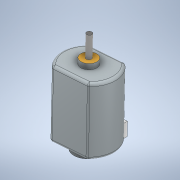
# Autodesk Inventor part: motor
Saved by Autodesk Inventor 2022 (Build 260153000, 153)
## iProperties
Created: 2022-06-21
Part Number: motor
Material: Generisch
Document SubType Name: Modeling
Designer: Friedrich Walmrath
Density: 1 g/cm^3
Appearance: Zink
Author: Friedrich Walmrath
Autodesk Inventor part; units mm, degrees
ref_plane "YZ Plane" through (0, 0, 0) normal (1, 0, 0) x (0, 1, 0)
ref_plane "XZ Plane" through (0, 0, 0) normal (0, 1, 0) x (-1, 0, 0)
ref_plane "XY Plane" through (0, 0, 0) normal (0, 0, 1) x (1, 0, 0)
sketch "Skizze1" plane through (0, 0, 0) normal (0, 0, 1) x (1, 0, 0)
  circle A0 centre (0, 0) radius 10
  line L0 (-6.6144, 7.5) -> (6.6144, 7.5)
  line L1 (-6.6144, -7.5) -> (6.6144, -7.5)
  dimension "d0" = 20
  dimension "d1" = 15
  constraints: 4 end point, 4 point on circle, 2 vertical alignment, 1 centre point, 1 coincident, 1 horizontal, 1 parallel
  measures "d0" diameter of A0
  measures "d1" distance between parallel lines of L1 L0
extrude "Extrusion1" add sketch "Skizze1" along normal blind 25 contours A0 L1 L0
sketch "Skizze2" plane through (0, 0, 25) normal (0, 0, 1) x (1, 0, 0)
  circle A0 centre (0, 0) radius 3
  dimension "d5" = 6
  constraints: 1 centre point, 1 coincident
  measures "d5" diameter of A0
extrude "Extrusion2" add sketch "Skizze2" along normal blind 2
sketch "Skizze3" plane through (0, 0, 27) normal (0, 0, 1) x (1, 0, 0)
  circle A0 centre (0, 0) radius 1
  dimension "d8" = 2
  constraints: 1 centre point, 1 coincident
  measures "d8" diameter of A0
extrude "Extrusion3" add sketch "Skizze3" along normal blind 8
sketch "Skizze5" plane through (-6.6144, 7.5, 0) normal (0, 1, 0) x (1, 0, 0)
  line L0 (0, 0) -> (13.2288, 0)
  line L1 (13.2288, 0) -> (13.2288, -5)
  line L2 (13.2288, -5) -> (0, -5)
  line L3 (0, -5) -> (0, 0)
  line L4 (13.2288, 0) -> (13.2288, -25) projected
  line L5 (0, 0) -> (0, -25) projected
  line L6 (13.2288, 0) -> (0, 0) projected
  point P0 (6.6144, 0)
  point P1 (13.2288, -2.5)
  point P2 (0, -2.5)
  dimension "d11" = 5
  constraints: 8 end point, 3 point on line, 2 midpoint, 2 parallel, 1 horizontal, 1 perpendicular
  measures "d11" distance between parallel lines of L2 L0
extrude "Extrusion4" add sketch "Skizze5" along normal blind 1.5
sketch "Skizze6" plane through (0, 0, 0) normal (0, 0, -1) x (-1, 0, 0)
  circle A0 centre (0, 0) radius 1 projected
  circle A1 centre (0, 0) radius 5
  dimension "d14" = 10
  constraints: 1 centre point, 1 coincident
  measures "d14" diameter of A1
extrude "Extrusion5" add sketch "Skizze6" along normal blind 2.75 contours A0 | A1
fillet "Rundung2" radius 1 11 edges at (0, -7.5, 25) (-6.6144, -7.5, 12.5) (-10, 0, 25) (0, 7.5, 25) (10, 0, 25) (6.6144, -7.5, 12.5) (6.6144, 7.5, 15) (10, 0, 0) (-10, 0, 0) (-6.6144, 7.5, 15) (0, -7.5, 0)
